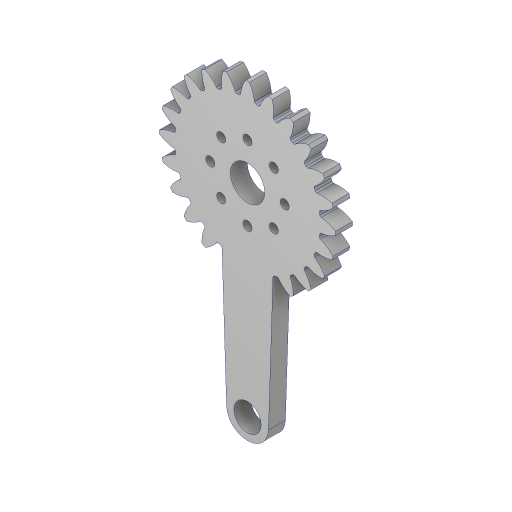
# Autodesk Inventor part: Gear(PCD 48, MOD 2)
Saved by Autodesk Inventor 2023.2 (Build 272271000, 271)
## iProperties
Created: 2021-07-28
Part Number: Gear(PCD 48, MOD 2)
Material: 알루미늄 6061
Document SubType Name: Modeling
Designer: user
Density: 2.7 g/cm^3
Appearance: 알루미늄 - 평지
Mass: 29.1582 g
Surface Area: 67.2047 cm^2
Volume: 10.7993 cm^3
Author: user
Autodesk Inventor part; units mm, degrees
ref_plane "YZ Plane" through (0, 0, 0) normal (1, 0, 0) x (0, 1, 0)
ref_plane "XZ Plane" through (0, 0, 0) normal (0, 1, 0) x (-1, 0, 0)
ref_plane "XY Plane" through (0, 0, 0) normal (0, 0, 1) x (1, 0, 0)
sketch "스케치1" plane through (0, 0, 0) normal (0, 0, 1) x (1, 0, 0)
  arc A0 (1.57, 23.9486) -> (-1.57, 23.9486) centre (0, 0) ccw
  arc A1 (-2.07, 21.4001) -> (2.07, 21.4001) centre (0, 0) ccw
  line L0 (0, 0) -> (0, 26)
  line L1 (-1.57, 0) -> (-1.57, 23.9486)
  line L2 (-0.57, 0) -> (-0.57, 25.9938)
  line L3 (-2.07, 0) -> (-2.07, 21.4001)
  arc A2 (-0.57, 25.9938) -> (-2.07, 21.4001) centre (7.2779, 20.8894) ccw
  line L4 (1.57, 0) -> (1.57, 23.9486)
  line L5 (0.57, 0) -> (0.57, 25.9938)
  line L6 (2.07, 0) -> (2.07, 21.4001)
  arc A3 (2.07, 21.4001) -> (0.57, 25.9938) centre (-7.2779, 20.8894) ccw
  arc A4 (0.57, 25.9938) -> (-0.57, 25.9938) centre (0, 0) ccw
  point P0 (-1.57, 29)
  point P1 (-0.57, 29)
  point P2 (-2.07, 29)
  point P3 (1.57, 29)
  point P4 (0.57, 29)
  point P5 (2.07, 29)
  dimension "d0" = 48
  dimension "d2" = 43
  dimension "d3" = 1.57
  dimension "d4" = 1
  dimension "d7" = 0.5
  constraints: 14 end point, 13 point on circle, 9 symmetric about line, 5 centre point, 3 coincident, 3 parallel, 1 vertical, 1 other
  measures "d0" diameter of A0
  measures "d2" diameter of A1
  measures "d3" distance between parallel lines of L0 L1
  measures "d4" distance between parallel lines of L1 L2
  measures "d7" distance between parallel lines of L3 L1
extrude "돌출1" add sketch "스케치1" along normal blind 5
sketch "스케치6" plane through (0, 0, 5) normal (0, 0, 1) x (1, 0, 0)
  circle A0 centre (0, -60) radius 4.025 projected
  circle A1 centre (0, -60) radius 4.8
  point P0 (0, 0)
  dimension "d42" = 9.6
  constraints: 1 centre point, 1 coincident
  measures "d42" diameter of A1
pattern_circular "원형 패턴1" count 24 over 360 about axis through (0, 0, 0) along (0, 0, 1) of "돌출1"
sketch "스케치2" plane through (0, 0, 5) normal (0, 0, 1) x (1, 0, 0)
  circle A0 centre (0, 0) radius 5.1
  line L0 (0, 0) -> (11, 0)
  line L1 (0, 0) -> (11, 0) construction
  circle A1 centre (11, 0) radius 1.35
  circle A2 centre (7.7782, 7.7782) radius 1.35
  circle A3 centre (0, 11) radius 1.35
  circle A4 centre (-7.7782, 7.7782) radius 1.35
  circle A5 centre (-11, 0) radius 1.35
  circle A6 centre (-7.7782, -7.7782) radius 1.35
  circle A7 centre (0, -11) radius 1.35
  circle A8 centre (7.7782, -7.7782) radius 1.35
  dimension "d13" = 10.2
  dimension "d14" = 11
  dimension "d15" = 0
  dimension "d16" = 2.7
  dimension "d19" = 360
  constraints: 9 centre point, 4 end point, 2 coincident, 2 horizontal, 1 collinear, 17 other
  measures "d13" diameter of A0
  measures "d14" distance of L0.start L0.end
  measures "d15" distance between parallel lines of L0 L1
  measures "d16" diameter of A1
extrude "돌출2" cut sketch "스케치2" against normal up to surface (5 mm away)
sketch "스케치3" plane through (0, 0, 5) normal (0, 0, 1) x (1, 0, 0)
  circle A0 centre (0, 0) radius 21.5
  arc A1 (-7.5382, -20.1352) -> (-7.2783, -24.9605) centre (1.6233, -22.0613) ccw projected
  arc A2 (-7.2783, -24.9605) -> (-6.1771, -25.2556) centre (0, 0) ccw projected
  arc A3 (-6.1771, -25.2556) -> (-3.5393, -21.2067) centre (-12.4365, -18.2939) ccw projected
  arc A4 (-2.07, -21.4001) -> (-0.57, -25.9938) centre (7.2779, -20.8894) ccw projected
  arc A5 (-0.57, -25.9938) -> (0.57, -25.9938) centre (0, 0) ccw projected
  arc A6 (0.57, -25.9938) -> (2.07, -21.4001) centre (-7.2779, -20.8894) ccw projected
  arc A7 (3.5393, -21.2067) -> (6.1771, -25.2556) centre (12.4365, -18.2939) ccw projected
  arc A8 (6.1771, -25.2556) -> (7.2783, -24.9605) centre (0, 0) ccw projected
  arc A9 (7.2783, -24.9605) -> (7.5382, -20.1352) centre (-1.6233, -22.0613) ccw projected
  dimension "d23" = 43
  constraints: 1 centre point, 1 coincident
  measures "d23" diameter of A0
extrude "돌출3" cut sketch "스케치3" against normal up to surface (5 mm away) contours A0 A3 A2 A1 | A9 A8 A7 A0 | A0 A6 A5 A4
sketch "스케치4" plane through (0, 0, 5) normal (0, 0, 1) x (1, 0, 0)
  circle A0 centre (0, 0) radius 21.5
  line L0 (0, 0) -> (0, -66)
  line L1 (0, 0) -> (66, 0) construction
  line L2 (0, -66) -> (6, -66)
  arc A1 (7.5382, -20.1352) -> (8.9074, -19.568) centre (0, 0) ccw projected
  line L3 (6, -66) -> (7.5382, -20.1352)
  line L4 (0, -66) -> (-6, -66)
  line L5 (0, -66) -> (6, -66) construction
  arc A2 (-7.5382, -20.1352) -> (-7.2783, -24.9605) centre (1.6233, -22.0613) ccw projected
  line L6 (-6, -66) -> (-7.5382, -20.1352)
  dimension "d26" = 43
  dimension "d27" = 66
  dimension "d28" = 90
  dimension "d29" = 6
  dimension "d30" = 90
  dimension "d31" = 6
  dimension "d32" = 180
  constraints: 14 end point, 3 horizontal, 2 equal length, 1 centre point, 1 coincident, 1 perpendicular, 1 vertical
  measures "d26" diameter of A0
  measures "d27" distance of L0.start L0.end
  measures "d28" angle of L0 L1
  measures "d29" distance of L0.end L2.end
  measures "d30" angle of L2 L0
  measures "d31" distance of L0.end L4.end
  measures "d32" angle of L4 L5
extrude "돌출4" add sketch "스케치4" against normal up to surface (5 mm away) contours A0 L0 L4 L6 | A0 L3 L2 L0
fillet "모깎기1" radius 0.5 44 edges at (7.5382, -20.1352, 2.5) (8.9074, -19.568, 2.5) (12.4927, -17.498, 2.5) (13.6685, -16.5959, 2.5) (17.498, -12.4927, 2.5) (20.1352, -7.5382, 2.5) (21.4001, -2.07, 2.5) (16.5959, -13.6685, 2.5) (19.568, -8.9074, 2.5) (21.2067, -3.5393, 2.5) (21.2067, 3.5393, 2.5) (21.4001, 2.07, 2.5) (19.568, 8.9074, 2.5) (16.5959, 13.6685, 2.5) (12.4927, 17.498, 2.5) (7.5382, 20.1352, 2.5) (20.1352, 7.5382, 2.5) (17.498, 12.4927, 2.5) (13.6685, 16.5959, 2.5) (8.9074, 19.568, 2.5) (3.5393, 21.2067, 2.5) (2.07, 21.4001, 2.5) (-3.5393, 21.2067, 2.5) (-2.07, 21.4001, 2.5) (-8.9074, 19.568, 2.5) (-7.5382, 20.1352, 2.5) (-13.6685, 16.5959, 2.5) (-17.498, 12.4927, 2.5) (-20.1352, 7.5382, 2.5) (-12.4927, 17.498, 2.5) (-16.5959, 13.6685, 2.5) (-19.568, 8.9074, 2.5) (-21.4001, 2.07, 2.5) (-21.2067, -3.5393, 2.5) (-21.2067, 3.5393, 2.5) (-21.4001, -2.07, 2.5) (-19.568, -8.9074, 2.5) (-20.1352, -7.5382, 2.5) (-17.498, -12.4927, 2.5) (-16.5959, -13.6685, 2.5) (-13.6685, -16.5959, 2.5) (-12.4927, -17.498, 2.5) (-8.9074, -19.568, 2.5) (-7.5382, -20.1352, 2.5)
fillet "모깎기2" radius 6 2 edges at (6, -66, 2.5) (-6, -66, 2.5)
sketch "스케치5" plane through (0, 0, 5) normal (0, 0, 1) x (1, 0, 0)
  line L0 (0, -66) -> (0, -60)
  line L1 (0, -66) -> (6, -66) construction
  line L2 (-0.1979, -66) -> (0.1979, -66) projected
  circle A0 centre (0, -60) radius 4.025
  point P0 (0, 0)
  point P1 (0, -66)
  dimension "d37" = 6
  dimension "d38" = 90
  dimension "d39" = 8.05
  constraints: 4 end point, 2 perpendicular, 1 centre point, 1 coincident, 1 horizontal, 1 midpoint, 1 point on line, 1 vertical
  measures "d37" distance of L0.start L0.end
  measures "d38" angle of L1 L0
  measures "d39" diameter of A0
extrude "돌출5" cut sketch "스케치5" against normal up to surface (5 mm away)
